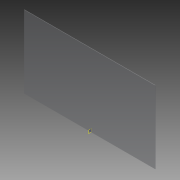
# Autodesk Inventor part: GE-13059
Saved by Autodesk Inventor 2013 (Build 170138000, 138)
## iProperties
Created: 2013-01-03
Part Number: GE-13059
Material: Polycarbonate, Clear
Document SubType Name: Modeling
Designer: Phillip
Density: 1 g/cm^3
Author: Phillip
Autodesk Inventor part; units mm, degrees
ref_plane "YZ Plane" through (0, 0, 0) normal (1, 0, 0) x (0, 1, 0)
ref_plane "XZ Plane" through (0, 0, 0) normal (0, 1, 0) x (-1, 0, 0)
ref_plane "XY Plane" through (0, 0, 0) normal (0, 0, 1) x (1, 0, 0)
sketch "Sketch1" plane through (0, 0, 0) normal (0, 0, 1) x (1, 0, 0)
  line L0 (-504.825, -279.4) -> (504.825, -279.4)
  line L1 (504.825, -279.4) -> (504.825, 279.4)
  line L2 (504.825, 279.4) -> (-504.825, 279.4)
  line L3 (-504.825, 279.4) -> (-504.825, -279.4)
  line L4 (-504.825, -279.4) -> (504.825, 279.4) construction
  line L5 (504.825, -279.4) -> (-504.825, 279.4) construction
  point P0 (0, 0)
  dimension "d0" = 1009.65
  dimension "d1" = 558.8
  constraints: 12 end point, 2 midpoint, 2 parallel, 1 horizontal, 1 perpendicular
  measures "d0" distance of L2.end L1.end
  measures "d1" distance of L1.end L0.end
extrude "Extrusion1" add sketch "Sketch1" against normal blind 3.175
ref_plane "Work Plane1" through (0, -279.4, -3.175) normal (-1, 0, 0) x (0, -1, 0)
body "Solid1"
